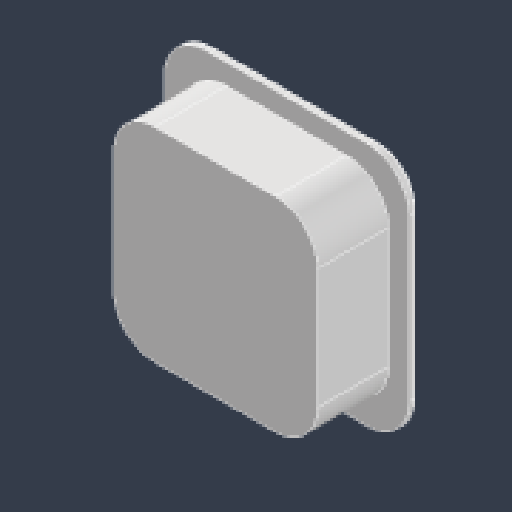
# Autodesk Inventor part: Speaker Cover
Saved by Autodesk Inventor 2023.4 (Build 274418000, 418)
## iProperties
Created: 2024-02-24
Part Number: Speaker Cover
Material: Generic
Document SubType Name: Modeling
Designer: JoaoSilva
Density: 1 g/cm^3
Appearance: Default
Author: JoaoSilva
Autodesk Inventor part; units mm, degrees
ref_plane "YZ Plane" through (0, 0, 0) normal (1, 0, 0) x (0, 1, 0)
ref_plane "XZ Plane" through (0, 0, 0) normal (0, 1, 0) x (-1, 0, 0)
ref_plane "XY Plane" through (0, 0, 0) normal (0, 0, 1) x (1, 0, 0)
sketch "Sketch1" plane through (0, 0, 0) normal (0, 0, 1) x (1, 0, 0)
  line L0 (-12, 12) -> (12, 12)
  line L1 (12, 12) -> (12, -12)
  line L2 (12, -12) -> (-12, -12)
  line L3 (-12, -12) -> (-12, 12)
  line L4 (-12, 12) -> (12, -12) construction
  line L5 (12, 12) -> (-12, -12) construction
  point P0 (0, 0)
  dimension "d0" = 24
  dimension "d1" = 24
  constraints: 12 end point, 2 midpoint, 2 parallel, 1 horizontal, 1 perpendicular
  measures "d0" distance of L1.end L2.end
  measures "d1" distance of L0.end L1.end
extrude "Extrusion1" add sketch "Sketch1" along normal blind 1
sketch "Sketch2" plane through (0, 0, 1) normal (0, 0, 1) x (1, 0, 0)
  line L0 (-10, 10) -> (10, 10)
  line L1 (10, 10) -> (10, -10)
  line L2 (10, -10) -> (-10, -10)
  line L3 (-10, -10) -> (-10, 10)
  line L4 (-10, 10) -> (10, -10) construction
  line L5 (10, 10) -> (-10, -10) construction
  point P0 (0, 0)
  dimension "d4" = 20
  dimension "d5" = 20
  constraints: 12 end point, 2 midpoint, 2 parallel, 1 horizontal, 1 perpendicular
  measures "d4" distance of L1.end L2.end
  measures "d5" distance of L0.end L1.end
extrude "Extrusion2" add sketch "Sketch2" along normal blind 7
fillet "Fillet1" radius 4.1 8 edges at (10, 10, 4.5) (-10, 10, 4.5) (-10, -10, 4.5) (10, -10, 4.5) (12, -12, 0.5) (12, 12, 0.5) (-12, 12, 0.5) (-12, -12, 0.5)
chamfer "Chamfer1" distance 0.4 angle 45 8 edges at (-12, 0, 0) (-10.7991, -10.7991, 0) (0, -12, 0) (10.7991, -10.7991, 0) (12, 0, 0) (10.7991, 10.7991, 0) (0, 12, 0) (-10.7991, 10.7991, 0)
equation "\"d1\" = d0"
body "Solid1"
